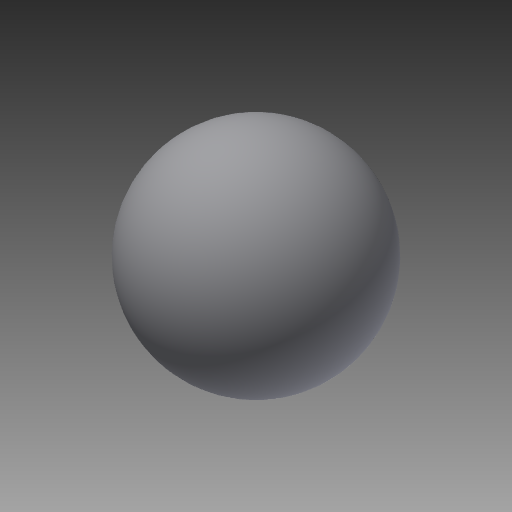
# Autodesk Inventor part: W 637/4 X-2Z_PART3
Saved by Autodesk Inventor 2019.1 (Build 231200000, 200)
## iProperties
Category: PARTsolutions
Company: SKF
Created: 2018-08-12
Part Number: W 637/4 X-2Z_PART3
Material: Allgemein
Catalog Web Link: www.cadenas.de
Description: -Deep groove ball bearings, stainless steel, single row
Vendor: SKF
Document SubType Name: Modeling
Designer: psadmin
Manufacturer: SKF
Mass: 0.000904779 g
Surface Area: 0.0452389 cm^2
Volume: 0.000904779 cm^3
Density: 1 g/cm^3
Appearance: PSOLRGB-192-192-192
PSOL_IDENT_0: {$CADENAS_DATA\23d-libs\skf\bearings_units_and_housings\ball_bearings\deep_groove_ball_bearings\deep
PSOL_IDENT_1: _groove_ball_bearings_stainless_steel\bb1_004_104.prj},203 {VTYP=3D},{NB=W 637/4 X-2Z_PART3},{LINA=W
PSOL_IDENT_2: 637/4 X-2Z_PART3},{NN=BB1_004_104_PART3},{NOPRJ=TRUE},{DATE=13.07.2018 14:28:03},{GEOMDATE=26.07.20
PSOL_IDENT_3: 17 12:34:56},{VERSION=},{LINEID=77400},{WBVAR=},{WBNUMERIC=}  {NB=W 637/4 X-2Z_PART3},{LINA=W 637/4
PSOL_IDENT_4: X-2Z_PART3},{KT=DUMMY},{PRODUCTID=},{DESIGNATION=W 637/4 X-2Z},{DD=4.000},{D=8.000},{B=3.000},{DD1=5
PSOL_IDENT_5: .000},{DD2=MIN},{D1=6.800},{D2=7.400},{R12A=0.100},{LOAD1=0.225},{LOAD2=0.072},{LOAD3=0.003},{SPEED1=
PSOL_IDENT_6: 75000},{SPEED2=},{MASS=0.001},{PITCH=5.900},{DW=1.200},{Z=7.000},{II=1.000},{TYPEID=MIN},{YALG=2.5},
PSOL_IDENT_7: {HALG=0.5},{HELP=0.6},{HELP2=0.3},{YALG1=3.4},{HALG1=0.6},{TAXONOMY=2},{DESIGN=dgbbw2z},{MAPPING=BCZ
PSOL_IDENT_8: 50,DESIGNATION|IRD01,DD|ORD10,D|BCW30,B|IRD30,DD1|ORD30,D1|ORD43,D2|IRD43,DD2|ORR20,R12A|BCC02,LOAD1
PSOL_IDENT_9: |BCC16,LOAD2|BCC12,LOAD3|BCC45,SPEED1|BCM01,MASS|BCD50,PITCH|RBD10,DW|BCN81,Z|BCN80,II},{DESIGNLIST=
PSOL_IDENT_10: dgbbw2z,dgbbw,dgbbw2rs},{SH=2.5},{SORT=DD},{RHELP=0.1},{PIM=W 637/4 X-2Z},{R12=0.1},{HIDE=MIN}
NT: Deep groove ball bearings, stainless steel, single row
NB: W 637/4 X-2Z_PART3
NBSYN: $DESIGNATION._PART3
LINA: W 637/4 X-2Z_PART3
SUPPLIER: SKF
ARTICLENO: W 637/4 X-2Z_PART3
BOMINFO: W 637/4 X-2Z_PART3
CREATOR: CADENAS GmbH
Title: W 637/4 X-2Z_PART3
Author: Cadenas PARTsolutions
Comments: Deep groove ball bearings, stainless steel, single row
Autodesk Inventor part; units mm, degrees
ref_plane "YZ Plane" through (0, 0, 0) normal (1, 0, 0) x (0, 1, 0)
ref_plane "XZ Plane" through (0, 0, 0) normal (0, 1, 0) x (-1, 0, 0)
ref_plane "XY Plane" through (0, 0, 0) normal (0, 0, 1) x (1, 0, 0)
sketch "Sketch_3" plane through (0, 0, 0) normal (0, 0, 1) x (1, 0, 0)
  line L0 (2.1, 2.95) -> (0.9, 2.95)
  arc A0 (2.1, 2.95) -> (0.9, 2.95) centre (1.5, 2.95) ccw
  line L1 (2.1, 2.95) -> (0.9, 2.95)
  dimension "d0" = 360
  constraints: 4 end point, 2 point on circle, 1 centre point
revolve "Revolution1" add sketch "Sketch_3" angle 360 about axis through (2.1, 2.95, 0) along (1, 0, 0)
body "Solid1"
